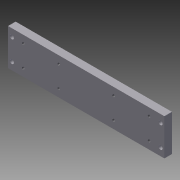
# Autodesk Inventor part: MagnetPlate
Saved by Autodesk Inventor 2012 (Build 160160000, 160)
## iProperties
Created: 2012-04-08
Part Number: MagnetPlate
Material: Aluminum-6061
Document SubType Name: Modeling
Designer: admin
Density: 2.71 g/cm^3
Mass: 226.967 g
Surface Area: 235.011 cm^2
Volume: 83.7517 cm^3
Author: admin
Autodesk Inventor part; units mm, degrees
ref_plane "YZ Plane" through (0, 0, 0) normal (1, 0, 0) x (0, 1, 0)
ref_plane "XZ Plane" through (0, 0, 0) normal (0, 1, 0) x (-1, 0, 0)
ref_plane "XY Plane" through (0, 0, 0) normal (0, 0, 1) x (1, 0, 0)
sketch "Sketch1" plane through (0, 0, 0) normal (0, 0, 1) x (1, 0, 0)
  line L0 (0, 0) -> (195.58, 0)
  line L1 (195.58, 0) -> (195.58, 45.72)
  line L2 (195.58, 45.72) -> (0, 45.72)
  line L3 (0, 45.72) -> (0, 0)
  dimension "d0" = 45.72
  dimension "d1" = 195.58
  constraints: 8 end point, 2 parallel, 1 horizontal, 1 perpendicular
  measures "d0" distance of L2.end L0.start
  measures "d1" distance of L0.start L0.end
extrude "Extrusion1" add sketch "Sketch1" along normal blind 9.525
sketch "Sketch2" plane through (0, 0, 0) normal (0, 0, -1) x (-1, 0, 0)
  circle A0 centre (-176.53, 36.195) radius 4.4323 projected
  circle A1 centre (-132.08, 36.195) radius 4.4323 projected
  circle A2 centre (-132.08, 9.525) radius 4.4323 projected
  circle A3 centre (-176.53, 9.525) radius 4.4323 projected
  circle A4 centre (-63.5, 36.195) radius 4.4323 projected
  circle A5 centre (-19.05, 36.195) radius 4.4323 projected
  circle A6 centre (-19.05, 9.525) radius 4.4323 projected
  circle A7 centre (-63.5, 9.525) radius 4.4323 projected
  constraints: 8 coincident
hole "Hole1" at (176.53, 36.195, 0) at (132.08, 36.195, 0) at (132.08, 9.525, 0) at (176.53, 9.525, 0) at (63.5, 9.525, 0) at (63.5, 36.195, 0) at (19.05, 36.195, 0) at (19.05, 9.525, 0) direction (0, 0, 1) diameter 3.302 end through all thread size "8-32 UNC" class "2B" standard "ANSI Unified Screw Threads"
sketch "Sketch3" plane through (0, 0, 0) normal (0, 0, -1) x (-1, 0, 0)
  circle A0 centre (-19.05, 9.525) radius 1.651 projected
  circle A1 centre (-19.05, 36.195) radius 1.651 projected
  line L0 (-195.58, 46.9392) -> (-195.58, -0.0508)
  line L1 (-186.055, -0.0508) -> (-195.58, -0.0508)
  line L2 (-186.055, -0.0508) -> (-186.055, 46.9392)
  line L3 (-195.58, 46.9392) -> (-186.055, 46.9392)
  line L4 (0, 46.9392) -> (0, -0.0508)
  line L5 (0, 46.9392) -> (-9.525, 46.9392)
  line L6 (-9.525, -0.0508) -> (-9.525, 46.9392)
  line L7 (-9.525, -0.0508) -> (0, -0.0508)
  circle A2 centre (-4.7625, 36.195) radius 1.651
  circle A3 centre (-4.7625, 9.525) radius 1.651
  line L8 (-195.58, 45.72) -> (0, 45.72) projected
  point P0 (-4.7625, 9.525)
  point P1 (-4.7625, 36.195)
  point P2 (-190.8175, 36.195)
  point P3 (-190.8175, 9.525)
  dimension "d18" = 9.525
  constraints: 16 end point, 2 centre point
  measures "d18" distance from line of L8 point (-4.762, 36.195)
hole "Hole2" at (4.7625, 9.525, 0) at (4.7625, 36.195, 0) at (190.8175, 36.195, 0) at (190.8175, 9.525, 0) direction (0, 0, 1) diameter 4.4958 end through all countersink diameter 8.4328 countersink angle 82 clearance for "Flat Head Machine Screw (82)" size "#8" standard "Ansi Unified Screw Threads"
body "Solid1"
